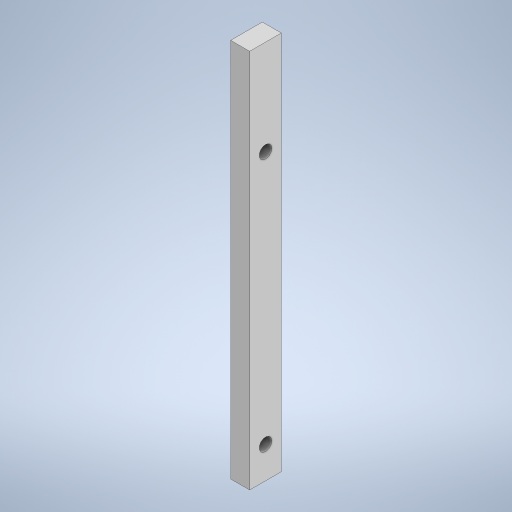
# Autodesk Inventor part: support
Saved by Autodesk Inventor 2023 (Build 270158000, 158)
## iProperties
Created: 2022-06-05
Part Number: support
Material: Generic
Document SubType Name: Modeling
Designer: prana_p9lsmih
Density: 1 g/cm^3
Appearance: Default
Author: prana_p9lsmih
Autodesk Inventor part; units mm, degrees
ref_plane "YZ Plane" through (0, 0, 0) normal (1, 0, 0) x (0, 1, 0)
ref_plane "XZ Plane" through (0, 0, 0) normal (0, 1, 0) x (-1, 0, 0)
ref_plane "XY Plane" through (0, 0, 0) normal (0, 0, 1) x (1, 0, 0)
sketch "Sketch1" plane through (0, 0, 0) normal (1, 0, 0) x (0, 1, 0)
  line L0 (0, 0) -> (60, 0)
  line L1 (60, 0) -> (60, 5)
  line L2 (60, 5) -> (0, 5)
  line L3 (0, 5) -> (0, 0)
  dimension "d0" = 60
  dimension "d1" = 5
  constraints: 8 end point, 3 perpendicular, 1 horizontal
  measures "d0" distance of L0.start L0.end
  measures "d1" distance of L0.end L1.end
extrude "Extrusion1" add sketch "Sketch1" along normal blind 3
sketch "Sketch2" plane through (3, 0, 0) normal (1, 0, 0) x (0, 0, -1)
  line L0 (-5, 0) -> (0, 0) projected
  line L1 (-5, 60) -> (-5, 0) projected
  point P0 (-2.5, 5)
  dimension "d4" = 5
  dimension "d5" = 2.5
  measures "d4" distance from line of L0 point (-2.5, 5)
  measures "d5" distance from line of L1 point (-2.5, 5)
hole "Hole1" at (3, 5, 2.5) direction (-1, 0, 0) diameter 2 end through all
sketch "Sketch3" plane through (3, 0, 0) normal (1, 0, 0) x (0, 0, -1)
  line L0 (-5, 0) -> (0, 0) projected
  line L1 (-5, 60) -> (-5, 0) projected
  point P0 (-2.5, 45)
  dimension "d13" = 45
  dimension "d14" = 2.5
  measures "d13" distance from line of L0 point (-2.5, 45)
  measures "d14" distance from line of L1 point (-2.5, 45)
hole "Hole2" at (3, 45, 2.5) direction (-1, 0, 0) diameter 2 end through all
body "Solid1"
